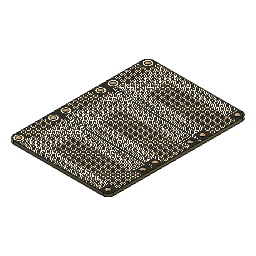
3417 Tripler FeatherWing (Autodesk Fusion 360 design; units mm, degrees)
part number: FEATHERWING_NODIM
Autodesk Fusion 360 part; units mm, degrees
sketch "sketch 305" plane through (0, 0, 0) normal (0, 0, 1) x (1, 0, 0)
  line L0 (0, 2.54) -> (0, 68.58)
  arc A0 (2.54, 71.12) -> (0, 68.58) centre (2.54, 68.58) ccw
  line L1 (2.54, 71.12) -> (48.26, 71.12)
  arc A1 (50.8, 68.58) -> (48.26, 71.12) centre (48.26, 68.58) ccw
  line L2 (50.8, 68.58) -> (50.8, 2.54)
  arc A2 (48.26, 0) -> (50.8, 2.54) centre (48.26, 2.54) ccw
  line L3 (48.26, 0) -> (2.54, 0)
  arc A3 (0, 2.54) -> (2.54, 0) centre (2.54, 2.54) ccw
extrude "Board" add sketch "sketch 305" along normal blind 1.57 makes body 1 in component "Board"
sketch "sketch 3589" plane through (0, 0, 0) normal (0, 0, 1) x (1, 0, 0)
  line L0 (0, 0) -> (50.8, 0)
  line L1 (50.8, 0) -> (50.8, 22.86)
  line L2 (50.8, 22.86) -> (0, 22.86)
  line L3 (0, 22.86) -> (0, 0)
extrude "FEATHERWING_DIM" add sketch "sketch 3589" along normal blind 0.1 separate body makes body 2 in component "FEATHERWING_DIM"
sketch "sketch 3737" plane through (0, 0, 0) normal (0, 0, 1) x (1, 0, 0)
  line L0 (-19.55, -0.5) -> (19.55, -0.5)
  line L1 (19.55, -0.5) -> (19.55, 0.5)
  line L2 (19.55, 0.5) -> (-19.55, 0.5)
  line L3 (-19.55, 0.5) -> (-19.55, -0.5)
extrude "1X16_ROUND_76MIL" add sketch "sketch 3737" along normal blind 0.1 separate body makes body 3 in component "1X16_ROUND_76MIL"
sketch "sketch 3885" plane through (0, 0, 0) normal (0, 0, 1) x (1, 0, 0)
  line L0 (-15.24, -0.635) -> (14.47, -0.635)
  line L1 (14.47, -0.635) -> (14.47, 0.635)
  line L2 (14.47, 0.635) -> (-15.24, 0.635)
  line L3 (-15.24, 0.635) -> (-15.24, -0.635)
extrude "1X12_ROUND_76MIL" add sketch "sketch 3885" along normal blind 0.1 separate body makes body 4 in component "1X12_ROUND_76MIL"
sketch "sketch 7199" plane through (0, 0, 0) normal (0, 0, 1) x (1, 0, 0)
  circle A0 centre (13.97, 6.35) radius 0.55
  circle A1 centre (13.97, 8.89) radius 0.55
  circle A2 centre (13.97, 11.43) radius 0.55
  circle A3 centre (13.97, 13.97) radius 0.55
  circle A4 centre (13.97, 16.51) radius 0.55
  circle A5 centre (13.97, 19.05) radius 0.55
  circle A6 centre (13.97, 21.59) radius 0.55
  circle A7 centre (13.97, 45.72) radius 0.55
  circle A8 centre (13.97, 43.18) radius 0.55
  circle A9 centre (13.97, 40.64) radius 0.55
  circle A10 centre (13.97, 38.1) radius 0.55
  circle A11 centre (13.97, 35.56) radius 0.55
  circle A12 centre (13.97, 33.02) radius 0.55
  circle A13 centre (13.97, 30.48) radius 0.55
  circle A14 centre (13.97, 69.85) radius 0.55
  circle A15 centre (13.97, 67.31) radius 0.55
  circle A16 centre (13.97, 64.77) radius 0.55
  circle A17 centre (13.97, 62.23) radius 0.55
  circle A18 centre (13.97, 59.69) radius 0.55
  circle A19 centre (13.97, 57.15) radius 0.55
  circle A20 centre (13.97, 54.61) radius 0.55
  circle A21 centre (8.89, 6.35) radius 0.55
  circle A22 centre (8.89, 8.89) radius 0.55
  circle A23 centre (8.89, 11.43) radius 0.55
  circle A24 centre (8.89, 13.97) radius 0.55
  circle A25 centre (8.89, 16.51) radius 0.55
  circle A26 centre (8.89, 19.05) radius 0.55
  circle A27 centre (8.89, 21.59) radius 0.55
  circle A28 centre (8.89, 30.48) radius 0.55
  circle A29 centre (8.89, 33.02) radius 0.55
  circle A30 centre (8.89, 35.56) radius 0.55
  circle A31 centre (8.89, 38.1) radius 0.55
  circle A32 centre (8.89, 40.64) radius 0.55
  circle A33 centre (8.89, 43.18) radius 0.55
  circle A34 centre (8.89, 45.72) radius 0.55
  circle A35 centre (8.89, 54.61) radius 0.55
  circle A36 centre (8.89, 57.15) radius 0.55
  circle A37 centre (8.89, 59.69) radius 0.55
  circle A38 centre (8.89, 62.23) radius 0.55
  circle A39 centre (8.89, 64.77) radius 0.55
  circle A40 centre (8.89, 67.31) radius 0.55
  circle A41 centre (8.89, 69.85) radius 0.55
  circle A42 centre (6.35, 6.35) radius 0.55
  circle A43 centre (11.43, 6.35) radius 0.55
  circle A44 centre (11.43, 8.89) radius 0.55
  circle A45 centre (6.35, 8.89) radius 0.55
  circle A46 centre (6.35, 11.43) radius 0.55
  circle A47 centre (3.81, 6.35) radius 0.55
  circle A48 centre (1.27, 6.35) radius 0.55
  circle A49 centre (1.27, 8.89) radius 0.55
  circle A50 centre (3.81, 8.89) radius 0.55
  circle A51 centre (3.81, 11.43) radius 0.55
  circle A52 centre (1.27, 11.43) radius 0.55
  circle A53 centre (1.27, 13.97) radius 0.55
  circle A54 centre (3.81, 13.97) radius 0.55
  circle A55 centre (6.35, 13.97) radius 0.55
  circle A56 centre (11.43, 13.97) radius 0.55
  circle A57 centre (11.43, 11.43) radius 0.55
  circle A58 centre (1.27, 16.51) radius 0.55
  circle A59 centre (3.81, 16.51) radius 0.55
  circle A60 centre (6.35, 16.51) radius 0.55
  circle A61 centre (11.43, 16.51) radius 0.55
  circle A62 centre (11.43, 21.59) radius 0.55
  circle A63 centre (11.43, 19.05) radius 0.55
  circle A64 centre (6.35, 21.59) radius 0.55
  circle A65 centre (6.35, 19.05) radius 0.55
  circle A66 centre (16.51, 6.35) radius 0.55
  circle A67 centre (16.51, 8.89) radius 0.55
  circle A68 centre (16.51, 11.43) radius 0.55
  circle A69 centre (16.51, 13.97) radius 0.55
  circle A70 centre (16.51, 16.51) radius 0.55
  circle A71 centre (19.05, 16.51) radius 0.55
  circle A72 centre (19.05, 13.97) radius 0.55
  circle A73 centre (19.05, 11.43) radius 0.55
  circle A74 centre (19.05, 8.89) radius 0.55
  circle A75 centre (19.05, 6.35) radius 0.55
  circle A76 centre (21.59, 6.35) radius 0.55
  circle A77 centre (21.59, 8.89) radius 0.55
  circle A78 centre (21.59, 11.43) radius 0.55
  circle A79 centre (21.59, 13.97) radius 0.55
  circle A80 centre (21.59, 16.51) radius 0.55
  circle A81 centre (24.13, 16.51) radius 0.55
  circle A82 centre (24.13, 13.97) radius 0.55
  circle A83 centre (24.13, 11.43) radius 0.55
  circle A84 centre (24.13, 8.89) radius 0.55
  circle A85 centre (24.13, 6.35) radius 0.55
  circle A86 centre (26.67, 6.35) radius 0.55
  circle A87 centre (26.67, 8.89) radius 0.55
  circle A88 centre (26.67, 11.43) radius 0.55
  circle A89 centre (26.67, 13.97) radius 0.55
  circle A90 centre (26.67, 16.51) radius 0.55
  circle A91 centre (29.21, 16.51) radius 0.55
  circle A92 centre (29.21, 13.97) radius 0.55
  circle A93 centre (29.21, 11.43) radius 0.55
  circle A94 centre (29.21, 8.89) radius 0.55
  circle A95 centre (29.21, 6.35) radius 0.55
  circle A96 centre (31.75, 6.35) radius 0.55
  circle A97 centre (34.29, 6.35) radius 0.55
  circle A98 centre (36.83, 6.35) radius 0.55
  circle A99 centre (39.37, 6.35) radius 0.55
  circle A100 centre (41.91, 6.35) radius 0.55
  circle A101 centre (41.91, 8.89) radius 0.55
  circle A102 centre (41.91, 11.43) radius 0.55
  circle A103 centre (41.91, 13.97) radius 0.55
  circle A104 centre (41.91, 16.51) radius 0.55
  circle A105 centre (39.37, 16.51) radius 0.55
  circle A106 centre (39.37, 13.97) radius 0.55
  circle A107 centre (39.37, 11.43) radius 0.55
  circle A108 centre (39.37, 8.89) radius 0.55
  circle A109 centre (36.83, 8.89) radius 0.55
  circle A110 centre (36.83, 11.43) radius 0.55
  circle A111 centre (36.83, 13.97) radius 0.55
  circle A112 centre (36.83, 16.51) radius 0.55
  circle A113 centre (34.29, 16.51) radius 0.55
  circle A114 centre (34.29, 13.97) radius 0.55
  circle A115 centre (34.29, 11.43) radius 0.55
  circle A116 centre (34.29, 8.89) radius 0.55
  circle A117 centre (31.75, 8.89) radius 0.55
  circle A118 centre (31.75, 11.43) radius 0.55
  circle A119 centre (31.75, 13.97) radius 0.55
  circle A120 centre (31.75, 16.51) radius 0.55
  circle A121 centre (44.45, 16.51) radius 0.55
  circle A122 centre (44.45, 13.97) radius 0.55
  circle A123 centre (44.45, 11.43) radius 0.55
  circle A124 centre (44.45, 8.89) radius 0.55
  circle A125 centre (44.45, 6.35) radius 0.55
  circle A126 centre (46.99, 6.35) radius 0.55
  circle A127 centre (49.53, 6.35) radius 0.55
  circle A128 centre (49.53, 8.89) radius 0.55
  circle A129 centre (46.99, 8.89) radius 0.55
  circle A130 centre (46.99, 11.43) radius 0.55
  circle A131 centre (49.53, 11.43) radius 0.55
  circle A132 centre (49.53, 13.97) radius 0.55
  circle A133 centre (46.99, 13.97) radius 0.55
  circle A134 centre (46.99, 16.51) radius 0.55
  circle A135 centre (49.53, 16.51) radius 0.55
  circle A136 centre (44.45, 30.48) radius 0.55
  circle A137 centre (44.45, 33.02) radius 0.55
  circle A138 centre (44.45, 35.56) radius 0.55
  circle A139 centre (44.45, 38.1) radius 0.55
  circle A140 centre (44.45, 40.64) radius 0.55
  circle A141 centre (41.91, 40.64) radius 0.55
  circle A142 centre (41.91, 38.1) radius 0.55
  circle A143 centre (41.91, 35.56) radius 0.55
  circle A144 centre (41.91, 33.02) radius 0.55
  circle A145 centre (41.91, 30.48) radius 0.55
  circle A146 centre (46.99, 30.48) radius 0.55
  circle A147 centre (46.99, 33.02) radius 0.55
  circle A148 centre (46.99, 35.56) radius 0.55
  circle A149 centre (46.99, 38.1) radius 0.55
  circle A150 centre (46.99, 40.64) radius 0.55
  circle A151 centre (49.53, 40.64) radius 0.55
  circle A152 centre (49.53, 38.1) radius 0.55
  circle A153 centre (49.53, 35.56) radius 0.55
  circle A154 centre (49.53, 33.02) radius 0.55
  circle A155 centre (49.53, 30.48) radius 0.55
  circle A156 centre (39.37, 30.48) radius 0.55
  circle A157 centre (39.37, 33.02) radius 0.55
  circle A158 centre (39.37, 35.56) radius 0.55
  circle A159 centre (39.37, 38.1) radius 0.55
  circle A160 centre (39.37, 40.64) radius 0.55
  circle A161 centre (36.83, 40.64) radius 0.55
  circle A162 centre (36.83, 38.1) radius 0.55
  circle A163 centre (36.83, 35.56) radius 0.55
  circle A164 centre (36.83, 33.02) radius 0.55
  circle A165 centre (36.83, 30.48) radius 0.55
  circle A166 centre (34.29, 30.48) radius 0.55
  circle A167 centre (34.29, 33.02) radius 0.55
  circle A168 centre (34.29, 35.56) radius 0.55
  circle A169 centre (34.29, 38.1) radius 0.55
  circle A170 centre (34.29, 40.64) radius 0.55
  circle A171 centre (31.75, 40.64) radius 0.55
  circle A172 centre (31.75, 38.1) radius 0.55
  circle A173 centre (31.75, 35.56) radius 0.55
  circle A174 centre (31.75, 33.02) radius 0.55
  circle A175 centre (31.75, 30.48) radius 0.55
  circle A176 centre (29.21, 30.48) radius 0.55
  circle A177 centre (29.21, 33.02) radius 0.55
  circle A178 centre (29.21, 35.56) radius 0.55
  circle A179 centre (29.21, 38.1) radius 0.55
  circle A180 centre (29.21, 40.64) radius 0.55
  circle A181 centre (26.67, 40.64) radius 0.55
  circle A182 centre (26.67, 38.1) radius 0.55
  circle A183 centre (26.67, 35.56) radius 0.55
  circle A184 centre (26.67, 33.02) radius 0.55
  circle A185 centre (26.67, 30.48) radius 0.55
  circle A186 centre (24.13, 30.48) radius 0.55
  circle A187 centre (24.13, 33.02) radius 0.55
  circle A188 centre (24.13, 35.56) radius 0.55
  circle A189 centre (24.13, 38.1) radius 0.55
  circle A190 centre (24.13, 40.64) radius 0.55
  circle A191 centre (21.59, 40.64) radius 0.55
  circle A192 centre (21.59, 38.1) radius 0.55
  circle A193 centre (21.59, 35.56) radius 0.55
  circle A194 centre (21.59, 33.02) radius 0.55
  circle A195 centre (21.59, 30.48) radius 0.55
  circle A196 centre (19.05, 30.48) radius 0.55
  circle A197 centre (19.05, 33.02) radius 0.55
  circle A198 centre (19.05, 35.56) radius 0.55
  circle A199 centre (19.05, 38.1) radius 0.55
  circle A200 centre (19.05, 40.64) radius 0.55
  circle A201 centre (16.51, 40.64) radius 0.55
  circle A202 centre (16.51, 38.1) radius 0.55
  circle A203 centre (16.51, 35.56) radius 0.55
  circle A204 centre (16.51, 33.02) radius 0.55
  circle A205 centre (16.51, 30.48) radius 0.55
  circle A206 centre (11.43, 30.48) radius 0.55
  circle A207 centre (11.43, 33.02) radius 0.55
  circle A208 centre (11.43, 35.56) radius 0.55
  circle A209 centre (11.43, 38.1) radius 0.55
  circle A210 centre (11.43, 40.64) radius 0.55
  circle A211 centre (11.43, 43.18) radius 0.55
  circle A212 centre (11.43, 45.72) radius 0.55
  circle A213 centre (6.35, 30.48) radius 0.55
  circle A214 centre (6.35, 33.02) radius 0.55
  circle A215 centre (6.35, 35.56) radius 0.55
  circle A216 centre (6.35, 38.1) radius 0.55
  circle A217 centre (6.35, 40.64) radius 0.55
  circle A218 centre (6.35, 43.18) radius 0.55
  circle A219 centre (6.35, 45.72) radius 0.55
  circle A220 centre (3.81, 40.64) radius 0.55
  circle A221 centre (1.27, 40.64) radius 0.55
  circle A222 centre (1.27, 38.1) radius 0.55
  circle A223 centre (3.81, 38.1) radius 0.55
  circle A224 centre (3.81, 35.56) radius 0.55
  circle A225 centre (1.27, 35.56) radius 0.55
  circle A226 centre (1.27, 33.02) radius 0.55
  circle A227 centre (3.81, 33.02) radius 0.55
  circle A228 centre (3.81, 30.48) radius 0.55
  circle A229 centre (1.27, 30.48) radius 0.55
  circle A230 centre (44.45, 54.61) radius 0.55
  circle A231 centre (44.45, 57.15) radius 0.55
  circle A232 centre (44.45, 59.69) radius 0.55
  circle A233 centre (44.45, 62.23) radius 0.55
  circle A234 centre (44.45, 64.77) radius 0.55
  circle A235 centre (41.91, 64.77) radius 0.55
  circle A236 centre (41.91, 62.23) radius 0.55
  circle A237 centre (41.91, 59.69) radius 0.55
  circle A238 centre (41.91, 57.15) radius 0.55
  circle A239 centre (41.91, 54.61) radius 0.55
  circle A240 centre (46.99, 54.61) radius 0.55
  circle A241 centre (46.99, 57.15) radius 0.55
  circle A242 centre (46.99, 59.69) radius 0.55
  circle A243 centre (46.99, 62.23) radius 0.55
  circle A244 centre (46.99, 64.77) radius 0.55
  circle A245 centre (49.53, 64.77) radius 0.55
  circle A246 centre (49.53, 62.23) radius 0.55
  circle A247 centre (49.53, 59.69) radius 0.55
  circle A248 centre (49.53, 57.15) radius 0.55
  circle A249 centre (49.53, 54.61) radius 0.55
  circle A250 centre (39.37, 54.61) radius 0.55
  circle A251 centre (39.37, 57.15) radius 0.55
  circle A252 centre (39.37, 59.69) radius 0.55
  circle A253 centre (39.37, 62.23) radius 0.55
  circle A254 centre (39.37, 64.77) radius 0.55
  circle A255 centre (36.83, 64.77) radius 0.55
  circle A256 centre (36.83, 62.23) radius 0.55
  circle A257 centre (36.83, 59.69) radius 0.55
  circle A258 centre (36.83, 57.15) radius 0.55
  circle A259 centre (36.83, 54.61) radius 0.55
  circle A260 centre (34.29, 54.61) radius 0.55
  circle A261 centre (34.29, 57.15) radius 0.55
  circle A262 centre (34.29, 59.69) radius 0.55
  circle A263 centre (34.29, 62.23) radius 0.55
  circle A264 centre (34.29, 64.77) radius 0.55
  circle A265 centre (31.75, 64.77) radius 0.55
  circle A266 centre (31.75, 62.23) radius 0.55
  circle A267 centre (31.75, 59.69) radius 0.55
  circle A268 centre (31.75, 57.15) radius 0.55
  circle A269 centre (31.75, 54.61) radius 0.55
  circle A270 centre (29.21, 54.61) radius 0.55
  circle A271 centre (29.21, 57.15) radius 0.55
  circle A272 centre (29.21, 59.69) radius 0.55
  circle A273 centre (29.21, 62.23) radius 0.55
  circle A274 centre (29.21, 64.77) radius 0.55
  circle A275 centre (26.67, 64.77) radius 0.55
  circle A276 centre (26.67, 62.23) radius 0.55
  circle A277 centre (26.67, 59.69) radius 0.55
  circle A278 centre (26.67, 57.15) radius 0.55
  circle A279 centre (26.67, 54.61) radius 0.55
  circle A280 centre (24.13, 54.61) radius 0.55
  circle A281 centre (24.13, 57.15) radius 0.55
  circle A282 centre (24.13, 59.69) radius 0.55
  circle A283 centre (24.13, 62.23) radius 0.55
  circle A284 centre (24.13, 64.77) radius 0.55
  circle A285 centre (21.59, 64.77) radius 0.55
  circle A286 centre (21.59, 62.23) radius 0.55
  circle A287 centre (21.59, 59.69) radius 0.55
  circle A288 centre (21.59, 57.15) radius 0.55
  circle A289 centre (21.59, 54.61) radius 0.55
  circle A290 centre (19.05, 54.61) radius 0.55
  circle A291 centre (19.05, 57.15) radius 0.55
  circle A292 centre (19.05, 59.69) radius 0.55
  circle A293 centre (19.05, 62.23) radius 0.55
  circle A294 centre (19.05, 64.77) radius 0.55
  circle A295 centre (16.51, 64.77) radius 0.55
  circle A296 centre (16.51, 62.23) radius 0.55
  circle A297 centre (16.51, 59.69) radius 0.55
  circle A298 centre (16.51, 57.15) radius 0.55
  circle A299 centre (16.51, 54.61) radius 0.55
  circle A300 centre (11.43, 54.61) radius 0.55
  circle A301 centre (11.43, 57.15) radius 0.55
  circle A302 centre (11.43, 59.69) radius 0.55
  circle A303 centre (11.43, 62.23) radius 0.55
  circle A304 centre (11.43, 64.77) radius 0.55
  circle A305 centre (11.43, 67.31) radius 0.55
  circle A306 centre (11.43, 69.85) radius 0.55
  circle A307 centre (6.35, 54.61) radius 0.55
  circle A308 centre (6.35, 57.15) radius 0.55
  circle A309 centre (6.35, 59.69) radius 0.55
  circle A310 centre (6.35, 62.23) radius 0.55
  circle A311 centre (6.35, 64.77) radius 0.55
  circle A312 centre (6.35, 67.31) radius 0.55
  circle A313 centre (6.35, 69.85) radius 0.55
  circle A314 centre (3.81, 64.77) radius 0.55
  circle A315 centre (1.27, 64.77) radius 0.55
  circle A316 centre (1.27, 62.23) radius 0.55
  circle A317 centre (3.81, 62.23) radius 0.55
  circle A318 centre (3.81, 59.69) radius 0.55
  circle A319 centre (1.27, 59.69) radius 0.55
  circle A320 centre (1.27, 57.15) radius 0.55
  circle A321 centre (3.81, 57.15) radius 0.55
  circle A322 centre (3.81, 54.61) radius 0.55
  circle A323 centre (1.27, 54.61) radius 0.55
  circle A324 centre (48.26, 20.32) radius 1.27
  circle A325 centre (48.26, 2.54) radius 1.27
  circle A326 centre (2.54, 20.32) radius 1.25
  circle A327 centre (2.54, 2.54) radius 1.25
  circle A328 centre (16.51, 21.59) radius 0.5
  circle A329 centre (19.05, 21.59) radius 0.5
  circle A330 centre (21.59, 21.59) radius 0.5
  circle A331 centre (24.13, 21.59) radius 0.5
  circle A332 centre (26.67, 21.59) radius 0.5
  circle A333 centre (29.21, 21.59) radius 0.5
  circle A334 centre (31.75, 21.59) radius 0.5
  circle A335 centre (34.29, 21.59) radius 0.5
  circle A336 centre (36.83, 21.59) radius 0.5
  circle A337 centre (39.37, 21.59) radius 0.5
  circle A338 centre (41.91, 21.59) radius 0.5
  circle A339 centre (44.45, 21.59) radius 0.5
  circle A340 centre (16.51, 1.27) radius 0.5
  circle A341 centre (19.05, 1.27) radius 0.5
  circle A342 centre (21.59, 1.27) radius 0.5
  circle A343 centre (24.13, 1.27) radius 0.5
  circle A344 centre (26.67, 1.27) radius 0.5
  circle A345 centre (29.21, 1.27) radius 0.5
  circle A346 centre (31.75, 1.27) radius 0.5
  circle A347 centre (34.29, 1.27) radius 0.5
  circle A348 centre (36.83, 1.27) radius 0.5
  circle A349 centre (39.37, 1.27) radius 0.5
  circle A350 centre (41.91, 1.27) radius 0.5
  circle A351 centre (44.45, 1.27) radius 0.5
  circle A352 centre (13.97, 1.27) radius 0.5
  circle A353 centre (11.43, 1.27) radius 0.5
  circle A354 centre (8.89, 1.27) radius 0.5
  circle A355 centre (6.35, 1.27) radius 0.5
  circle A356 centre (48.26, 44.45) radius 1.27
  circle A357 centre (48.26, 26.67) radius 1.27
  circle A358 centre (2.54, 44.45) radius 1.25
  circle A359 centre (2.54, 26.67) radius 1.25
  circle A360 centre (16.51, 45.72) radius 0.5
  circle A361 centre (19.05, 45.72) radius 0.5
  circle A362 centre (21.59, 45.72) radius 0.5
  circle A363 centre (24.13, 45.72) radius 0.5
  circle A364 centre (26.67, 45.72) radius 0.5
  circle A365 centre (29.21, 45.72) radius 0.5
  circle A366 centre (31.75, 45.72) radius 0.5
  circle A367 centre (34.29, 45.72) radius 0.5
  circle A368 centre (36.83, 45.72) radius 0.5
  circle A369 centre (39.37, 45.72) radius 0.5
  circle A370 centre (41.91, 45.72) radius 0.5
  circle A371 centre (44.45, 45.72) radius 0.5
  circle A372 centre (16.51, 25.4) radius 0.5
  circle A373 centre (19.05, 25.4) radius 0.5
  circle A374 centre (21.59, 25.4) radius 0.5
  circle A375 centre (24.13, 25.4) radius 0.5
  circle A376 centre (26.67, 25.4) radius 0.5
  circle A377 centre (29.21, 25.4) radius 0.5
  circle A378 centre (31.75, 25.4) radius 0.5
  circle A379 centre (34.29, 25.4) radius 0.5
  circle A380 centre (36.83, 25.4) radius 0.5
  circle A381 centre (39.37, 25.4) radius 0.5
  circle A382 centre (41.91, 25.4) radius 0.5
  circle A383 centre (44.45, 25.4) radius 0.5
  circle A384 centre (13.97, 25.4) radius 0.5
  circle A385 centre (11.43, 25.4) radius 0.5
  circle A386 centre (8.89, 25.4) radius 0.5
  circle A387 centre (6.35, 25.4) radius 0.5
  circle A388 centre (48.26, 68.58) radius 1.27
  circle A389 centre (48.26, 50.8) radius 1.27
  circle A390 centre (2.54, 68.58) radius 1.25
  circle A391 centre (2.54, 50.8) radius 1.25
  circle A392 centre (16.51, 69.85) radius 0.5
  circle A393 centre (19.05, 69.85) radius 0.5
  circle A394 centre (21.59, 69.85) radius 0.5
  circle A395 centre (24.13, 69.85) radius 0.5
  circle A396 centre (26.67, 69.85) radius 0.5
  circle A397 centre (29.21, 69.85) radius 0.5
  circle A398 centre (31.75, 69.85) radius 0.5
  circle A399 centre (34.29, 69.85) radius 0.5
  circle A400 centre (36.83, 69.85) radius 0.5
  circle A401 centre (39.37, 69.85) radius 0.5
  circle A402 centre (41.91, 69.85) radius 0.5
  circle A403 centre (44.45, 69.85) radius 0.5
  circle A404 centre (16.51, 49.53) radius 0.5
  circle A405 centre (19.05, 49.53) radius 0.5
  circle A406 centre (21.59, 49.53) radius 0.5
  circle A407 centre (24.13, 49.53) radius 0.5
  circle A408 centre (26.67, 49.53) radius 0.5
  circle A409 centre (29.21, 49.53) radius 0.5
  circle A410 centre (31.75, 49.53) radius 0.5
  circle A411 centre (34.29, 49.53) radius 0.5
  circle A412 centre (36.83, 49.53) radius 0.5
  circle A413 centre (39.37, 49.53) radius 0.5
  circle A414 centre (41.91, 49.53) radius 0.5
  circle A415 centre (44.45, 49.53) radius 0.5
  circle A416 centre (13.97, 49.53) radius 0.5
  circle A417 centre (11.43, 49.53) radius 0.5
  circle A418 centre (8.89, 49.53) radius 0.5
  circle A419 centre (6.35, 49.53) radius 0.5
  circle A420 centre (44.45, 3.81) radius 0.5
  circle A421 centre (41.91, 3.81) radius 0.5
  circle A422 centre (39.37, 3.81) radius 0.5
  circle A423 centre (36.83, 3.81) radius 0.5
  circle A424 centre (34.29, 3.81) radius 0.5
  circle A425 centre (31.75, 3.81) radius 0.5
  circle A426 centre (29.21, 3.81) radius 0.5
  circle A427 centre (26.67, 3.81) radius 0.5
  circle A428 centre (24.13, 3.81) radius 0.5
  circle A429 centre (21.59, 3.81) radius 0.5
  circle A430 centre (19.05, 3.81) radius 0.5
  circle A431 centre (16.51, 3.81) radius 0.5
  circle A432 centre (13.97, 3.81) radius 0.5
  circle A433 centre (11.43, 3.81) radius 0.5
  circle A434 centre (8.89, 3.81) radius 0.5
  circle A435 centre (6.35, 3.81) radius 0.5
  circle A436 centre (44.45, 27.94) radius 0.5
  circle A437 centre (41.91, 27.94) radius 0.5
  circle A438 centre (39.37, 27.94) radius 0.5
  circle A439 centre (36.83, 27.94) radius 0.5
  circle A440 centre (34.29, 27.94) radius 0.5
  circle A441 centre (31.75, 27.94) radius 0.5
  circle A442 centre (29.21, 27.94) radius 0.5
  circle A443 centre (26.67, 27.94) radius 0.5
  circle A444 centre (24.13, 27.94) radius 0.5
  circle A445 centre (21.59, 27.94) radius 0.5
  circle A446 centre (19.05, 27.94) radius 0.5
  circle A447 centre (16.51, 27.94) radius 0.5
  circle A448 centre (13.97, 27.94) radius 0.5
  circle A449 centre (11.43, 27.94) radius 0.5
  circle A450 centre (8.89, 27.94) radius 0.5
  circle A451 centre (6.35, 27.94) radius 0.5
  circle A452 centre (44.45, 52.07) radius 0.5
  circle A453 centre (41.91, 52.07) radius 0.5
  circle A454 centre (39.37, 52.07) radius 0.5
  circle A455 centre (36.83, 52.07) radius 0.5
  circle A456 centre (34.29, 52.07) radius 0.5
  circle A457 centre (31.75, 52.07) radius 0.5
  circle A458 centre (29.21, 52.07) radius 0.5
  circle A459 centre (26.67, 52.07) radius 0.5
  circle A460 centre (24.13, 52.07) radius 0.5
  circle A461 centre (21.59, 52.07) radius 0.5
  circle A462 centre (19.05, 52.07) radius 0.5
  circle A463 centre (16.51, 52.07) radius 0.5
  circle A464 centre (13.97, 52.07) radius 0.5
  circle A465 centre (11.43, 52.07) radius 0.5
  circle A466 centre (8.89, 52.07) radius 0.5
  circle A467 centre (6.35, 52.07) radius 0.5
  circle A468 centre (16.51, 19.05) radius 0.5
  circle A469 centre (19.05, 19.05) radius 0.5
  circle A470 centre (21.59, 19.05) radius 0.5
  circle A471 centre (24.13, 19.05) radius 0.5
  circle A472 centre (26.67, 19.05) radius 0.5
  circle A473 centre (29.21, 19.05) radius 0.5
  circle A474 centre (31.75, 19.05) radius 0.5
  circle A475 centre (34.29, 19.05) radius 0.5
  circle A476 centre (36.83, 19.05) radius 0.5
  circle A477 centre (39.37, 19.05) radius 0.5
  circle A478 centre (41.91, 19.05) radius 0.5
  circle A479 centre (44.45, 19.05) radius 0.5
  circle A480 centre (16.51, 43.18) radius 0.5
  circle A481 centre (19.05, 43.18) radius 0.5
  circle A482 centre (21.59, 43.18) radius 0.5
  circle A483 centre (24.13, 43.18) radius 0.5
  circle A484 centre (26.67, 43.18) radius 0.5
  circle A485 centre (29.21, 43.18) radius 0.5
  circle A486 centre (31.75, 43.18) radius 0.5
  circle A487 centre (34.29, 43.18) radius 0.5
  circle A488 centre (36.83, 43.18) radius 0.5
  circle A489 centre (39.37, 43.18) radius 0.5
  circle A490 centre (41.91, 43.18) radius 0.5
  circle A491 centre (44.45, 43.18) radius 0.5
  circle A492 centre (16.51, 67.31) radius 0.5
  circle A493 centre (19.05, 67.31) radius 0.5
  circle A494 centre (21.59, 67.31) radius 0.5
  circle A495 centre (24.13, 67.31) radius 0.5
  circle A496 centre (26.67, 67.31) radius 0.5
  circle A497 centre (29.21, 67.31) radius 0.5
  circle A498 centre (31.75, 67.31) radius 0.5
  circle A499 centre (34.29, 67.31) radius 0.5
  circle A500 centre (36.83, 67.31) radius 0.5
  circle A501 centre (39.37, 67.31) radius 0.5
  circle A502 centre (41.91, 67.31) radius 0.5
  circle A503 centre (44.45, 67.31) radius 0.5
extrude "Extrude4" cut sketch "sketch 7199" along normal blind 1.57 bodies 1 in component "Board"
component "PCB Component" placed x (1, 0, 0) y (0, 1, 0) z (0, 0, 1) at (0, 0, 0)
component "Board" placed x (1, 0, 0) y (0, 1, 0) z (0, 0, 1) at (0, 0, 0) in component "PCB Component"
component "FEATHERWING_DIM" placed x (1, 0, 0) y (0, 1, 0) z (0, 0, 1) at (0, 0, 1.57) in component "PCB Component"
component "FEATHERWING_DIM" placed x (1, 0, 0) y (0, 1, 0) z (0, 0, 1) at (0, 24.13, 1.57) in component "PCB Component"
component "FEATHERWING_DIM" placed x (1, 0, 0) y (0, 1, 0) z (0, 0, 1) at (0, 48.26, 1.57) in component "PCB Component"
component "1X16_ROUND_76MIL" placed x (-1, 0, 0) y (0, -1, 0) z (0, 0, 1) at (25.4, 3.81, 1.57) in component "PCB Component"
component "1X16_ROUND_76MIL" placed x (-1, 0, 0) y (0, -1, 0) z (0, 0, 1) at (25.4, 27.94, 1.57) in component "PCB Component"
component "1X16_ROUND_76MIL" placed x (-1, 0, 0) y (0, -1, 0) z (0, 0, 1) at (25.4, 52.07, 1.57) in component "PCB Component"
component "1X12_ROUND_76MIL" placed x (1, 0, 0) y (0, 1, 0) z (0, 0, 1) at (30.48, 19.05, 1.57) in component "PCB Component"
component "1X12_ROUND_76MIL" placed x (1, 0, 0) y (0, 1, 0) z (0, 0, 1) at (30.48, 43.18, 1.57) in component "PCB Component"
component "1X12_ROUND_76MIL" placed x (1, 0, 0) y (0, 1, 0) z (0, 0, 1) at (30.48, 67.31, 1.57) in component "PCB Component"
named bodies: "Board", "FEATHERWING_DIM", "1X16_ROUND_76MIL", "1X12_ROUND_76MIL"
